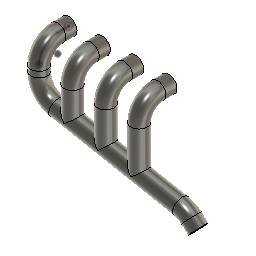
pipe attachment (Autodesk Fusion 360 design; units mm, degrees)
Autodesk Fusion 360 part; units mm, degrees
sketch "Sketch1" plane through (0, 0, 0) normal (1, 0, 0) x (0, 1, 0)
  line L0 (0, 0) -> (-30, 0)
  arc A0 (-30, 0) -> (-80, -50) centre (-30, -50) ccw
  dimension "d1" = 30
  dimension "d2" = 50
  dimension "d3" = 90
  constraint coincident L0.start origin
  constraint horizontal L0
  constraint tangent L0 A0
  measures "d1" distance of L0.start L0.end
  measures "d2" radius of A0
  measures "d3" angle of L0.end A0.end A0.centre
pipe "Pipe1" add diameter 45 wall 5 path "Sketch1" along A0 L0
ref_plane "WorkPlane1" through (0, -80, 0) normal (0, 1, 0) x (0, 0, 1)
sketch "Sketch2" plane through (0, -80, 0) normal (0, 1, 0) x (1, 0, 0)
  line L0 (0, 50) -> (0, 65.319934)
  arc A0 (48.637157, 124.234158) -> (0, 65.319934) centre (60, 65.319934) ccw
  line L1 (48.637157, 124.234158) -> (382.484426, 188.623604)
  arc A1 (382.484426, 188.623604) -> (411.513431, 203.170063) centre (371.121583, 247.537828) ccw
  line L2 (411.513431, 203.170063) -> (430, 220)
  line L3 (22.5, 50) -> (-22.5, 50)
  dimension "d9" = 15.319934
  dimension "d10" = 25
  dimension "d11" = 170
  dimension "d12" = 430
  dimension "d13" = 340
  dimension "d14" = 60
  constraint vertical L0
  constraint tangent L0 A0
  constraint tangent L1 A1
  constraint tangent A1 L2
  constraint tangent A0 L1
  constraint equal A0 A1
  constraint coincident L0.start L3
  constraint vertical origin L0.start
  measures "d11" vertical distance of L0.start L2.end
  measures "d12" horizontal distance of L0.start L2.end
  measures "d14" radius of A0
pipe "Pipe2" add diameter 45 wall 5 path "Sketch2" along L0 A0 L1 A1 L2
ref_plane "WorkPlane2" through (0, 0, -50) normal (0, 0, 1) x (1, 0, 0)
sketch "Sketch3" plane through (0, 0, -50) normal (0, 0, 1) x (1, 0, 0)
  circle A0 centre (90, -80) radius 22.5
  circle A1 centre (180, -80) radius 22.5
  circle A2 centre (270, -80) radius 22.5
  dimension "d20" = 45
  dimension "d21" = 90
  dimension "d22" = 80
  dimension "d25" = 90
  dimension "d26" = 0
  measures "d20" diameter of A0
  measures "d21" horizontal distance of origin A0.centre
  measures "d22" vertical distance of origin A0.centre
extrude "Extrude1" add sketch "Sketch3" along normal up to surface contours A0 | A1 | A2 picked at (96.757267, -83.254128) picked at (186.757267, -83.254128) picked at (275.248454, -75.991551) end surface at (155.679688, -77.759723, -167.680356)
sketch "Sketch4" plane through (0, 0, -50) normal (0, 0, 1) x (-1, 0, 0)
  circle A0 centre (-90, 80) radius 22.5
  circle A1 centre (-90, 80) radius 17.5
  circle A2 centre (-180, 80) radius 17.5
  circle A3 centre (-270, 80) radius 17.5
  dimension "d29" = 35
  dimension "d32" = -90
  dimension "d33" = 0
  constraint concentric A0 A1
  measures "d29" diameter of A1
extrude "Extrude2" cut sketch "Sketch4" along normal up to surface contours A1 | A2 | A3 picked at (-88.636808, 73.443507) picked at (-184.016977, 82.248269) picked at (-274.853818, 73.501337) end surface at (156.621886, -78.257563, -162.795234)
sweep "Sweep1" add 3 faces at (110.684411, -81.98723, -50) (200.684411, -81.98723, -50) (290.684411, -81.98723, -50) path "Sketch1" along L0 A0
